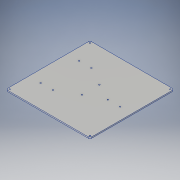
# Autodesk Inventor part: Heated Bed Plate
Saved by Autodesk Inventor 2020.3 (Build 243373000, 373)
## iProperties
Created: 2018-08-19
Part Number: Heated Bed Plate
Material: Aluminum 6061
Document SubType Name: Modeling
Designer: Richard
Density: 2.7 g/cm^3
Appearance: Aluminum - Flat
Author: Richard
Autodesk Inventor part; units mm, degrees
ref_plane "YZ Plane" through (0, 0, 0) normal (1, 0, 0) x (0, 1, 0)
ref_plane "XZ Plane" through (0, 0, 0) normal (0, 1, 0) x (-1, 0, 0)
ref_plane "XY Plane" through (0, 0, 0) normal (0, 0, 1) x (1, 0, 0)
sketch "Sketch1" plane through (0, 0, 0) normal (0, 1, 0) x (-1, 0, 0)
  line L0 (109.5, 109.5) -> (-109.5, 109.5)
  line L1 (-109.5, 109.5) -> (-109.5, -109.5)
  line L2 (-109.5, -109.5) -> (109.5, -109.5)
  line L3 (109.5, -109.5) -> (109.5, 109.5)
  line L4 (109.5, 109.5) -> (-109.5, -109.5) construction
  line L5 (-109.5, 109.5) -> (109.5, -109.5) construction
  point P0 (0, 0)
  dimension "d0" = 219
  constraints: 12 end point, 2 midpoint, 2 parallel, 2 perpendicular, 1 horizontal
  measures "d0" distance of L2.end L0.start
extrude "Extrusion1" add sketch "Sketch1" along normal mid plane 3.175
chamfer "Chamfer1" distance 4 angle 45 4 edges at (-109.5, 0, 109.5) (-109.5, 0, -109.5) (109.5, 0, -109.5) (109.5, 0, 109.5)
sketch "Sketch3" plane through (0, 1.5875, 0) normal (0, 1, 0) x (1, 0, 0)
  line L0 (-104.5, -104.5) -> (104.5, -104.5) construction
  line L1 (104.5, -104.5) -> (104.5, 104.5) construction
  line L2 (104.5, 104.5) -> (-104.5, 104.5) construction
  line L3 (-104.5, 104.5) -> (-104.5, -104.5) construction
  line L4 (-104.5, -104.5) -> (104.5, 104.5) construction
  line L5 (104.5, -104.5) -> (-104.5, 104.5) construction
  line L6 (-78.5, 50) -> (-46.5, 50) construction
  line L7 (-78.5, -50) -> (-46.5, -50) construction
  line L8 (46.5, 0) -> (78.5, 0) construction
  point P0 (0, 0)
  point P1 (0, 0)
  dimension "d16" = 209
  dimension "d17" = 209
  dimension "d18" = 32
  dimension "d20" = 46.5
  dimension "d21" = 46.5
  dimension "d22" = 100
  dimension "d23" = 50
  dimension "d24" = 93
  constraints: 18 end point, 10 coincident, 4 horizontal, 4 parallel, 3 midpoint, 1 perpendicular, 1 point on line, 1 vertical alignment
  measures "d16" distance of L2.end L1.end
  measures "d17" distance of L1.end L0.end
  measures "d18" distance of L6.start L6.end
  measures "d20" horizontal distance of point (0, 0) L6.end
  measures "d21" distance of L8.start point (0, 0)
  measures "d22" distance between parallel lines of L7 L6
  measures "d23" distance from line of point (0, 0) L6
  measures "d24" horizontal distance of L8.start L6.end
hole "Hole1" at (-104.5, 1.5875, -104.5) at (104.5, 1.5875, -104.5) at (104.5, 1.5875, 104.5) at (-104.5, 1.5875, 104.5) at (-78.5, 1.5875, -50) at (-46.5, 1.5875, -50) at (46.5, 1.5875, 0) at (78.5, 1.5875, 0) at (-46.5, 1.5875, 50) at (-78.5, 1.5875, 50) direction (0, -1, 0) diameter 3.2 end through all
sketch "Sketch4" plane through (0, 1.5875, 0) normal (0, 1, 0) x (1, 0, 0)
  line L0 (1.5, 22.5) -> (1.5, -22.5)
  line L1 (-109.5, 105.5) -> (-109.5, -105.5) projected
  point P0 (0, 0)
  point P1 (-114.5, 42.3569)
  point P2 (1.5, 0)
  point P3 (-109.5, -105.5)
  dimension "d38" = 45
  dimension "d39" = 111
  constraints: 2 coincident, 2 end point, 1 horizontal alignment, 1 midpoint, 1 vertical, 1 other
  measures "d38" distance of L0.start L0.end
hole "Hole2" at (1.5, 1.5875, -22.5) at (1.5, 1.5875, 22.5) direction (0, -1, 0) diameter 3.4036 depth 6.4 clearance for "Flat Head Machine Screw" size "M3" standard "Ansi Metric M Profile"
equation "\"d21\" = d20"
body "Solid1"
